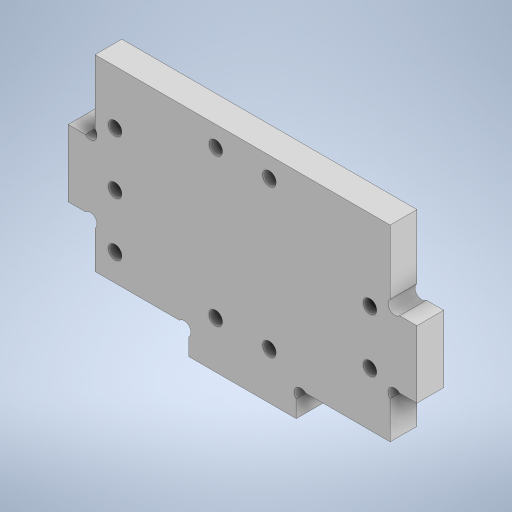
# Autodesk Inventor part: Front Wall
Saved by Autodesk Inventor 2023 (Build 270158000, 158)
## iProperties
Created: 2022-12-26
Part Number: Front Wall
Material: Generic
Document SubType Name: Modeling
Designer: justi
Density: 1 g/cm^3
Appearance: Default
Mass: 172.505 g
Surface Area: 360.429 cm^2
Volume: 172.505 cm^3
Author: justi
Autodesk Inventor part; units mm, degrees
ref_plane "YZ Plane" through (0, 0, 0) normal (1, 0, 0) x (0, 1, 0)
ref_plane "XZ Plane" through (0, 0, 0) normal (0, 1, 0) x (-1, 0, 0)
ref_plane "XY Plane" through (0, 0, 0) normal (0, 0, 1) x (1, 0, 0)
sketch "Sketch1" plane through (0, 0, 0) normal (0, 0, 1) x (1, 0, 0)
  line L0 (0, 0) -> (165.1, 0)
  line L1 (165.1, 0) -> (165.1, 101.6)
  line L2 (165.1, 101.6) -> (0, 101.6)
  line L3 (0, 101.6) -> (0, 0)
  line L4 (0, 0) -> (57.15, 0)
  line L5 (57.15, 0) -> (57.15, 12.7)
  line L6 (57.15, 12.7) -> (0, 12.7)
  line L7 (0, 12.7) -> (0, 0)
  line L8 (165.1, 0) -> (107.95, 0)
  line L9 (107.95, 0) -> (107.95, 12.7)
  line L10 (107.95, 12.7) -> (165.1, 12.7)
  line L11 (165.1, 12.7) -> (165.1, 0)
  line L12 (0, 12.7) -> (12.7, 12.7)
  line L13 (12.7, 12.7) -> (12.7, 34.925)
  line L14 (12.7, 34.925) -> (0, 34.925)
  line L15 (0, 34.925) -> (0, 12.7)
  line L16 (165.1, 12.7) -> (152.4, 12.7)
  line L17 (152.4, 12.7) -> (152.4, 34.925)
  line L18 (152.4, 34.925) -> (165.1, 34.925)
  line L19 (165.1, 34.925) -> (165.1, 12.7)
  line L20 (0, 101.6) -> (12.7, 101.6)
  line L21 (12.7, 101.6) -> (12.7, 66.675)
  line L22 (12.7, 66.675) -> (0, 66.675)
  line L23 (0, 66.675) -> (0, 101.6)
  line L24 (165.1, 101.6) -> (152.4, 101.6)
  line L25 (152.4, 101.6) -> (152.4, 66.675)
  line L26 (152.4, 66.675) -> (165.1, 66.675)
  line L27 (165.1, 66.675) -> (165.1, 101.6)
  point P0 (0, 66.675)
  point P1 (0, 34.925)
  dimension "d0" = 101.6
  dimension "d1" = 165.1
  dimension "d2" = 57.15
  dimension "d3" = 12.7
  dimension "d4" = 57.15
  dimension "d5" = 12.7
  dimension "d6" = 12.7
  dimension "d7" = 22.225
  dimension "d8" = 12.7
  dimension "d9" = 22.225
  dimension "d10" = 12.7
  dimension "d11" = 34.925
  dimension "d12" = 12.7
  dimension "d13" = 34.925
  constraints: 56 end point, 14 parallel, 7 horizontal, 7 perpendicular
  measures "d0" distance of L0.end L1.end
  measures "d1" distance of L1.end L2.end
  measures "d2" distance of L6.end L5.end
  measures "d3" distance of L4.end L5.end
  measures "d4" distance of L9.end L10.end
  measures "d5" distance of L8.end L9.end
  measures "d6" distance of L14.end L13.end
  measures "d7" distance of L12.end L13.end
  measures "d8" distance of L17.end L18.end
  measures "d9" distance of L16.end L17.end
  measures "d10" distance of L21.end L22.end
  measures "d11" distance of L20.end L21.end
  measures "d12" distance of L26.end L25.end
  measures "d13" distance of L24.end L25.end
extrude "Extrusion1" add sketch "Sketch1" along normal blind 12.7 contours L5 L6 L13 L14 L3 L22 L21 L2 L25 L26 L1 L18 L17 L10 L9 L0
sketch "Sketch2" plane through (0, 0, 12.7) normal (0, 0, 1) x (1, 0, 0)
  line L0 (12.7, 66.675) -> (0, 66.675) projected
  line L1 (12.7, 66.675) -> (10.4549, 68.9201)
  line L2 (12.7, 101.6) -> (12.7, 66.675) projected
  line L3 (12.7, 34.925) -> (12.7, 12.7) projected
  line L4 (12.7, 34.925) -> (10.4549, 32.6799)
  line L5 (57.15, 12.7) -> (57.15, 0) projected
  line L6 (57.15, 12.7) -> (54.9049, 10.4549)
  line L7 (107.95, 0) -> (107.95, 12.7) projected
  line L8 (107.95, 12.7) -> (110.1951, 10.4549)
  line L9 (107.95, 12.7) -> (152.4, 12.7) projected
  line L10 (152.4, 12.7) -> (152.4, 34.925) projected
  line L11 (152.4, 34.925) -> (154.6451, 32.6799)
  line L12 (152.4, 34.925) -> (165.1, 34.925) projected
  line L13 (165.1, 66.675) -> (152.4, 66.675) projected
  line L14 (152.4, 66.675) -> (154.6451, 68.9201)
  circle A0 centre (10.4549, 68.9201) radius 3.175
  circle A1 centre (10.4549, 32.6799) radius 3.175
  circle A2 centre (54.9049, 10.4549) radius 3.175
  circle A3 centre (110.1951, 10.4549) radius 3.175
  circle A4 centre (154.6451, 32.6799) radius 3.175
  circle A5 centre (154.6451, 68.9201) radius 3.175
  point P0 (0, 0)
  dimension "d16" = 3.175
  dimension "d17" = 45
  dimension "d18" = 3.175
  dimension "d19" = 45
  dimension "d20" = 3.175
  dimension "d21" = 45
  dimension "d22" = 3.175
  dimension "d23" = 45
  dimension "d24" = 3.175
  dimension "d25" = 45
  dimension "d26" = 3.175
  dimension "d27" = 45
  dimension "d28" = 6.35
  dimension "d29" = 6.35
  dimension "d30" = 6.35
  dimension "d31" = 6.35
  dimension "d32" = 6.35
  dimension "d33" = 6.35
  constraints: 12 end point, 6 centre point, 5 point on line
  measures "d16" distance of L0.start L1.end
  measures "d17" angle of L2 L1
  measures "d18" distance of L3.start L4.end
  measures "d19" angle of L3 L4
  measures "d20" distance of L5.start L6.end
  measures "d21" angle of L5 L6
  measures "d22" distance of L7.end L8.end
  measures "d23" angle of L9 L8
  measures "d24" distance of L10.end L11.end
  measures "d25" angle of L12 L11
  measures "d26" distance of L13.end L14.end
  measures "d27" angle of L13 L14
  measures "d28" diameter of A0
  measures "d29" diameter of A1
  measures "d30" diameter of A2
  measures "d31" diameter of A3
  measures "d32" diameter of A4
  measures "d33" diameter of A5
extrude "Extrusion2" cut sketch "Sketch2" against normal blind 12.7
sketch "Sketch4" plane through (0, 0, 12.7) normal (0, 0, 1) x (1, 0, 0)
  circle A0 centre (22.225, 82.55) radius 3.175
  circle A1 centre (22.225, 57.15) radius 3.175
  line L0 (12.7, 101.6) -> (12.7, 71.1651) projected
  circle A2 centre (22.225, 31.75) radius 3.175
  line L1 (12.7, 30.4349) -> (12.7, 12.7) projected
  line L2 (57.15, 0) -> (107.95, 0) projected
  circle A3 centre (142.875, 31.75) radius 3.175
  circle A4 centre (142.875, 57.15) radius 3.175
  circle A5 centre (142.875, 82.55) radius 3.175
  line L3 (152.4, 71.1651) -> (152.4, 101.6) projected
  line L4 (152.4, 12.7) -> (152.4, 30.4349) projected
  circle A6 centre (82.55, 22.225) radius 3.175
  line L5 (112.4401, 12.7) -> (152.4, 12.7) projected
  line L6 (57.15, 8.2099) -> (57.15, 0) projected
  circle A7 centre (57.15, 22.225) radius 3.175
  line L7 (12.7, 12.7) -> (52.6599, 12.7) projected
  circle A8 centre (107.95, 22.225) radius 3.175
  point P0 (0, 0)
  dimension "d63" = 6.35
  dimension "d64" = 6.35
  dimension "d65" = 9.525
  dimension "d66" = 9.525
  dimension "d67" = 6.35
  dimension "d68" = 9.525
  dimension "d69" = 31.75
  dimension "d70" = 25.4
  dimension "d71" = 25.4
  dimension "d72" = 6.35
  dimension "d73" = 6.35
  dimension "d74" = 6.35
  dimension "d75" = 9.525
  dimension "d76" = 9.525
  dimension "d77" = 9.525
  dimension "d78" = 31.75
  dimension "d79" = 25.4
  dimension "d80" = 25.4
  dimension "d81" = 6.35
  dimension "d82" = 9.525
  dimension "d83" = 25.4
  dimension "d84" = 6.35
  dimension "d85" = 9.525
  dimension "d86" = 25.4
  dimension "d87" = 6.35
  dimension "d88" = 25.4
  dimension "d89" = 9.525
  constraints: 9 centre point
  measures "d63" diameter of A0
  measures "d64" diameter of A1
  measures "d65" distance from line of L0 A0.centre
  measures "d66" distance from line of L0 A1.centre
  measures "d67" diameter of A2
  measures "d68" distance from line of L1 A2.centre
  measures "d69" distance from line of L2 A2.centre
  measures "d70" distance of A1.centre A2.centre
  measures "d71" distance of A0.centre A1.centre
  measures "d72" diameter of A3
  measures "d73" diameter of A4
  measures "d74" diameter of A5
  measures "d75" distance from line of L3 A5.centre
  measures "d76" distance from line of L3 A4.centre
  measures "d77" distance from line of L4 A3.centre
  measures "d78" distance from line of L2 A3.centre
  measures "d79" distance of A3.centre A4.centre
  measures "d80" distance of A5.centre A4.centre
  measures "d81" diameter of A6
  measures "d82" distance from line of L5 A6.centre
  measures "d83" distance from line of L6 A6.centre
  measures "d84" diameter of A7
  measures "d85" distance from line of L7 A7.centre
  measures "d86" distance of A6.centre A7.centre
  measures "d87" diameter of A8
  measures "d88" distance of A6.centre A8.centre
  measures "d89" distance from line of L5 A8.centre
extrude "Extrusion4" cut sketch "Sketch4" against normal blind 12.7
sketch "Sketch5" plane through (0, 0, 12.7) normal (0, 0, 1) x (1, 0, 0)
  circle A0 centre (22.225, 76.2) radius 3.175
  circle A1 centre (22.225, 82.55) radius 3.175 projected
  circle A2 centre (22.225, 50.8) radius 3.175
  circle A3 centre (22.225, 25.4) radius 3.175
  line L0 (12.7, 101.6) -> (12.7, 71.1651) projected
  point P0 (0, 0)
  dimension "d92" = 6.35
  dimension "d93" = 6.35
  dimension "d94" = 6.35
  dimension "d95" = 6.35
  dimension "d96" = 9.525
  dimension "d97" = 9.525
  dimension "d98" = 9.525
  dimension "d99" = 25.4
  dimension "d100" = 25.4
  constraints: 3 centre point
  measures "d92" diameter of A0
  measures "d93" distance of A1.centre A0.centre
  measures "d94" diameter of A2
  measures "d95" diameter of A3
  measures "d96" distance from line of L0 A0.centre
  measures "d97" distance from line of L0 A2.centre
  measures "d98" distance from line of L0 A3.centre
  measures "d99" distance of A0.centre A2.centre
  measures "d100" distance of A2.centre A3.centre
extrude "Extrusion5" cut sketch "Sketch5" against normal blind 12.7 contours A0 | A2 | A3
sketch "Sketch6" plane through (0, 0, 12.7) normal (0, 0, 1) x (1, 0, 0)
  circle A0 centre (22.225, 82.55) radius 3.175 projected
  circle A1 centre (22.225, 82.55) radius 3.175
  circle A2 centre (22.225, 57.15) radius 3.175 projected
  circle A3 centre (22.225, 57.15) radius 3.175
  circle A4 centre (22.225, 31.75) radius 3.175 projected
  circle A5 centre (22.225, 31.75) radius 3.175
  point P0 (0, 0)
  point P1 (22.225, 79.375)
  point P2 (22.225, 53.975)
  point P3 (22.225, 28.575)
  dimension "d103" = 6.35
  dimension "d104" = 6.35
  dimension "d105" = 6.35
  constraints: 3 centre point, 3 coincident, 3 vertical alignment
  measures "d103" diameter of A1
  measures "d104" diameter of A3
  measures "d105" diameter of A5
extrude "Extrusion6" add sketch "Sketch6" against normal blind 12.7
sketch "Sketch8" plane through (0, 0, 12.7) normal (0, 0, 1) x (1, 0, 0)
  circle A0 centre (142.875, 82.55) radius 3.175 projected
  circle A1 centre (142.875, 82.55) radius 3.175
  circle A2 centre (142.875, 57.15) radius 3.175 projected
  circle A3 centre (142.875, 57.15) radius 3.175
  circle A4 centre (142.875, 31.75) radius 3.175 projected
  circle A5 centre (142.875, 31.75) radius 3.175
  point P0 (0, 0)
  dimension "d116" = 6.35
  dimension "d117" = 6.35
  dimension "d118" = 6.35
  constraints: 3 centre point, 3 coincident
  measures "d116" diameter of A1
  measures "d117" diameter of A3
  measures "d118" diameter of A5
extrude "Extrusion8" add sketch "Sketch8" against normal blind 12.7
sketch "Sketch11" plane through (0, 0, 12.7) normal (0, 0, 1) x (1, 0, 0)
  circle A0 centre (69.85, 22.225) radius 3.175
  circle A1 centre (95.25, 22.225) radius 3.175
  line L0 (12.7, 12.7) -> (52.6599, 12.7) projected
  line L1 (112.4401, 12.7) -> (152.4, 12.7) projected
  line L2 (57.15, 8.2099) -> (57.15, 0) projected
  line L3 (107.95, 0) -> (107.95, 8.2099) projected
  point P0 (0, 0)
  dimension "d132" = 6.35
  dimension "d133" = 6.35
  dimension "d134" = 9.525
  dimension "d135" = 9.525
  dimension "d136" = 12.7
  dimension "d137" = 12.7
  constraints: 2 centre point
  measures "d132" diameter of A0
  measures "d133" diameter of A1
  measures "d134" distance from line of L0 A0.centre
  measures "d135" distance from line of L1 A1.centre
  measures "d136" distance from line of L2 A0.centre
  measures "d137" distance from line of L3 A1.centre
extrude "Extrusion10" cut sketch "Sketch11" against normal blind 12.7
sketch "Sketch12" plane through (0, 0, 12.7) normal (0, 0, 1) x (1, 0, 0)
  circle A0 centre (82.55, 22.225) radius 3.175 projected
  circle A1 centre (82.55, 22.225) radius 3.175
  circle A2 centre (57.15, 22.225) radius 3.175 projected
  circle A3 centre (57.15, 22.225) radius 3.175
  circle A4 centre (107.95, 22.225) radius 3.175 projected
  circle A5 centre (107.95, 22.225) radius 3.175
  point P0 (0, 0)
  dimension "d140" = 6.35
  dimension "d141" = 6.35
  dimension "d142" = 6.35
  constraints: 3 centre point, 3 coincident
  measures "d140" diameter of A1
  measures "d141" diameter of A3
  measures "d142" diameter of A5
extrude "Extrusion11" add sketch "Sketch12" against normal blind 12.7
sketch "Sketch13" plane through (0, 0, 12.7) normal (0, 0, 1) x (1, 0, 0)
  circle A0 centre (69.85, 92.075) radius 3.175
  circle A1 centre (95.25, 92.075) radius 3.175
  line L0 (152.4, 101.6) -> (12.7, 101.6) projected
  line L1 (57.15, 8.2099) -> (57.15, 0) projected
  point P0 (0, 0)
  dimension "d145" = 6.35
  dimension "d146" = 6.35
  dimension "d147" = 9.525
  dimension "d148" = 9.525
  dimension "d149" = 25.4
  dimension "d150" = 12.7
  constraints: 2 centre point
  measures "d145" diameter of A0
  measures "d146" diameter of A1
  measures "d147" distance from line of L0 A0.centre
  measures "d148" distance from line of L0 A1.centre
  measures "d149" distance of A0.centre A1.centre
  measures "d150" distance from line of L1 A0.centre
extrude "Extrusion12" cut sketch "Sketch13" against normal blind 12.7
sketch "Sketch14" plane through (0, 0, 12.7) normal (0, 0, 1) x (1, 0, 0)
  line L0 (57.15, 0) -> (107.95, 0) projected
  line L1 (152.4, 12.7) -> (152.4, 30.4349) projected
  circle A0 centre (142.875, 38.1) radius 3.175
  circle A1 centre (142.875, 63.5) radius 3.175
  point P0 (0, 0)
  dimension "d156" = 6.35
  dimension "d158" = 6.35
  dimension "d160" = 9.525
  dimension "d161" = 9.525
  dimension "d162" = 25.4
  dimension "d165" = 38.1
  constraints: 2 centre point
  measures "d156" diameter of A0
  measures "d158" diameter of A1
  measures "d160" distance from line of L1 A0.centre
  measures "d161" distance from line of L1 A1.centre
  measures "d162" distance of A0.centre A1.centre
  measures "d165" distance from line of L0 A0.centre
extrude "Extrusion13" cut sketch "Sketch14" against normal blind 12.7
body "Solid1"
